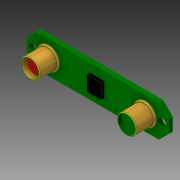
# Autodesk Inventor part: ZX_Distance_and_Gesture_Sensor_v10.brd_Outline
Saved by Autodesk Inventor 2016 SP1 (Build 200210100, 210)
## iProperties
Created: 2015-11-19
Part Number: ZX_Distance_and_Gesture_Sensor_v10.brd_Outline
Material: Generic
Document SubType Name: Modeling
Designer: PhillipD
Density: 1 g/cm^3
Appearance: Board Outline
Author: PhillipD
Autodesk Inventor part; units mm, degrees
ref_plane "YZ Plane" through (0, 0, 0) normal (1, 0, 0) x (0, 1, 0)
sketch "Sketch1" plane through (0, 0, 0) normal (0, 0, 1) x (1, 0, 0)
  line L0 (-24.13, 6.35) -> (24.13, 6.35)
  line L1 (24.13, 6.35) -> (27.94, 2.54)
  line L2 (27.94, 2.54) -> (27.94, -2.54)
  line L3 (27.94, -2.54) -> (24.13, -6.35)
  line L4 (24.13, -6.35) -> (-24.13, -6.35)
  line L5 (-24.13, -6.35) -> (-27.94, -2.54)
  line L6 (-27.94, -2.54) -> (-27.94, 2.54)
  line L7 (-27.94, 2.54) -> (-24.13, 6.35)
  circle A0 centre (-17.78, 0) radius 0.405
  circle A1 centre (-20.32, 0) radius 0.405
  circle A2 centre (17.78, 0) radius 0.405
  circle A3 centre (20.32, 0) radius 0.405
  circle A4 centre (-10.16, -5.08) radius 0.51
  circle A5 centre (-7.62, -5.08) radius 0.51
  circle A6 centre (-5.08, -5.08) radius 0.51
  circle A7 centre (-2.54, -5.08) radius 0.51
  circle A8 centre (0, -5.08) radius 0.51
  circle A9 centre (2.54, -5.08) radius 0.51
  circle A10 centre (5.08, -5.08) radius 0.51
  circle A11 centre (7.62, -5.08) radius 0.51
  circle A12 centre (10.16, -5.08) radius 0.51
  circle A13 centre (2.54, 5.08) radius 0.51
  circle A14 centre (0, 5.08) radius 0.51
  circle A15 centre (-2.54, 5.08) radius 0.51
  circle A16 centre (-25.4, 0) radius 1.651
  circle A17 centre (25.4, 0) radius 1.651
  circle A18 centre (6.223, -0.127) radius 0.1905
  circle A19 centre (5.1562, -2.3876) radius 0.1905
  circle A20 centre (21.844, -3.556) radius 0.1905
  circle A21 centre (-4.191, -2.413) radius 0.1905
  circle A22 centre (-11.938, -3.81) radius 0.1905
  circle A23 centre (-19.05, 2.6162) radius 0.1905
  circle A24 centre (-19.05, -2.032) radius 0.1905
  circle A25 centre (6.2484, -2.413) radius 0.1905
  circle A26 centre (6.35, -4.0894) radius 0.1905
  circle A27 centre (9.3472, 1.397) radius 0.1905
  circle A28 centre (13.97, 4.572) radius 0.1905
  circle A29 centre (19.05, 2.6162) radius 0.1905
  circle A30 centre (13.97, 0.889) radius 0.1905
  circle A31 centre (11.938, -5.08) radius 0.1905
  circle A32 centre (2.1082, -2.7432) radius 0.1905
  circle A33 centre (-11.43, 5.08) radius 0.1905
  circle A34 centre (-16.6116, -5.0546) radius 0.1905
  circle A35 centre (2.1336, 3.5052) radius 0.1905
  circle A36 centre (24.638, -3.81) radius 0.1905
  circle A37 centre (-24.638, 3.81) radius 0.1905
  circle A38 centre (-8.89, 5.08) radius 0.1905
  circle A39 centre (-8.8392, -2.9972) radius 0.1905
  circle A40 centre (4.2672, 4.7498) radius 0.1905
  circle A41 centre (3.81, -3.9878) radius 0.1905
  circle A42 centre (19.05, -2.2098) radius 0.1905
  circle A43 centre (-4.191, 2.4892) radius 0.1905
  circle A44 centre (-13.716, 3.556) radius 0.1905
  circle A45 centre (4.191, -0.127) radius 0.1905
  circle A46 centre (-11.43, -0.889) radius 0.1905
  circle A47 centre (4.191, 1.143) radius 0.1905
  circle A48 centre (-8.89, -0.889) radius 0.1905
  circle A49 centre (4.0386, -2.286) radius 0.1905
  circle A50 centre (0.0254, 2.6416) radius 0.1905
  circle A51 centre (8.89, 4.572) radius 0.1905
  circle A52 centre (-4.191, 0.8636) radius 0.1905
  circle A53 centre (-13.97, 4.826) radius 0.1905
  circle A54 centre (8.89, 3.302) radius 0.1905
  circle A55 centre (11.5316, 1.397) radius 0.1905
  circle A56 centre (-16.002, -3.4798) radius 0.1905
  circle A57 centre (-19.05, 4.572) radius 0.1905
  circle A58 centre (16.002, -3.556) radius 0.1905
  circle A59 centre (19.05, 4.572) radius 0.1905
  circle A60 centre (-7.239, 1.27) radius 0.1905
  circle A61 centre (0.7366, -2.54) radius 0.1905
  circle A62 centre (-0.381, -2.9972) radius 0.1905
  circle A63 centre (-7.7978, 3.7338) radius 0.1905
  circle A64 centre (-5.461, 1.27) radius 0.1905
  circle A65 centre (10.16, -2.54) radius 0.1905
  circle A66 centre (13.97, -0.889) radius 0.1905
  constraints: 67 centre point, 16 end point
extrude "ZX_Distance_and_Gesture_Sensor_v10.brd_Outline" add sketch "Sketch1" along normal blind 1.6
sketch "Sketch2" plane through (0, 0, 1.6) normal (0, 0, 1) x (1, 0, 0)
  line L0 (-28.8947, 7.8442) -> (28.2553, 7.8442) construction
  line L1 (28.2553, 7.8442) -> (28.2553, -7.7492) construction
  line L2 (28.2553, -7.7492) -> (-28.8947, -7.7492) construction
  line L3 (-28.8947, -7.7492) -> (-28.8947, 7.8442) construction
  circle A0 centre (-25.4, 0) radius 1.651 projected
  circle A1 centre (25.4, 0) radius 1.651 projected
  circle A2 centre (-19.05, 0.0475) radius 3.81
  circle A3 centre (-19.05, 0.0475) radius 3.429
  line L4 (-3.0061, 2.9488) -> (2.6936, 2.9488)
  line L5 (2.6936, 2.9488) -> (2.6936, -2.9972)
  line L6 (2.6936, -2.9972) -> (-3.0061, -2.9972)
  line L7 (-3.0061, -2.9972) -> (-3.0061, 2.9488)
  circle A4 centre (-20.32, 0) radius 0.405 projected
  circle A5 centre (-17.78, 0) radius 0.405 projected
  line L8 (-20.32, 0) -> (-17.78, 0) construction
  point P0 (0, 0)
  point P1 (-19.05, 0)
  dimension "d5" = 57.15
  dimension "d22" = 7.62
  dimension "d23" = 0.381
  constraints: 10 end point, 2 centre point, 2 horizontal, 2 parallel, 1 coincident, 1 midpoint, 1 perpendicular, 1 vertical alignment, 2 other
  measures "d5" distance between parallel lines of L1 L3
  measures "d22" diameter of A2
  measures "d23" radial gap between concentric circles of A2 A3
extrude "Extrusion2" add sketch "Sketch2" along normal blind 7.62 contours A2
extrude "Extrusion3" add sketch "Sketch2" along normal blind 6.0325 separate body contours A3 | A4 | A5
fillet "Fillet1" radius 0.254 1 edges at (-22.86, 0.0475, 9.22)
fillet "Fillet2" radius 1.27 1 edges at (-22.479, 0.0475, 7.6325)
ref_plane "Work Plane1" through (-19.05, 0.0475, 1.6) normal (0.7071, -0.7071, 0) x (0, 0, 1)
sketch "Sketch4" plane through (-19.05, 0.0475, 1.6) normal (0.7071, -0.7071, 0) x (0, 0, 1)
  line L0 (0, -3.81) -> (7.366, -3.81) projected
  line L1 (0.903, -3.81) -> (0.903, -3.9298)
  arc A0 (0, -4.1701) -> (0.903, -3.9298) centre (0.4195, -3.9298) ccw
  line L2 (0, 3.81) -> (0, -3.81) projected
  line L3 (0, -4.1701) -> (0, -3.81)
  line L4 (0, -3.81) -> (0.903, -3.81)
  line L5 (-3.444, 0) -> (9.464, 0) projected
  point P0 (-1.6, -13.4368)
  constraints: 6 end point, 2 perpendicular, 2 point on circle, 1 centre point, 1 collinear, 1 point on line, 1 tangent
revolve "Revolution1" add sketch "Sketch4" angle 360 about axis through (-19.05, 0.0475, 1.6) along (0, 0, 1) bodies 1
ref_plane "Work Plane2" through (0, 6.35, 1.6) normal (-1, 0, 0) x (0, -1, 0)
mirror "Mirror1" about plane through (0, 6.35, 1.6) normal (-1, 0, 0) of "Extrusion2" bodies 1
mirror "Mirror2" about plane through (0, 6.35, 1.6) normal (-1, 0, 0) of "Extrusion3" bodies 2
mirror "Mirror3" about plane through (0, 6.35, 1.6) normal (-1, 0, 0) of "Revolution1" bodies 1
extrude "Extrusion4" add sketch "Sketch2" along normal blind 1.27 contours L4 L5 L6 L7 bodies 1
sketch "Sketch5" plane through (0, 0, 1.6) normal (0, 0, 1) x (1, 0, 0)
  line L0 (-15.0069, 3.9379) -> (-3.3449, 3.9379) construction
  line L1 (-3.3449, 3.9379) -> (-3.3449, -3.9863) construction
  line L2 (-3.3449, -3.9863) -> (-15.0069, -3.9863) construction
  line L3 (-15.0069, -3.9863) -> (-15.0069, 3.9379) construction
  line L4 (-3.0061, 2.9488) -> (-3.0061, -2.9972) projected
  point P0 (0, 0)
  point P1 (-3.3449, -0.0242)
  point P2 (-3.0061, -0.0242)
  constraints: 2 midpoint, 1 horizontal alignment, 2 other
fillet "Fillet3" radius 0.254 1 edges at (22.86, 0.0475, 9.22)
body "Solid1"
body "Solid2"
